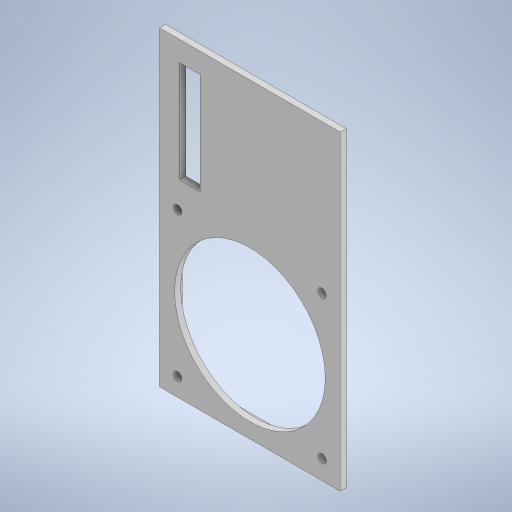
# Autodesk Inventor part: TapaControladora
Saved by Autodesk Inventor 2024 (Build 280153000, 153)
## iProperties
Created: 2023-11-28
Part Number: TapaControladora
Material: Genérico
Document SubType Name: Modeling
Designer: sergi
Density: 1 g/cm^3
Appearance: Valor por defecto
Author: sergi
Autodesk Inventor part; units mm, degrees
ref_plane "YZ Plane" through (0, 0, 0) normal (1, 0, 0) x (0, 1, 0)
ref_plane "XZ Plane" through (0, 0, 0) normal (0, 1, 0) x (-1, 0, 0)
ref_plane "XY Plane" through (0, 0, 0) normal (0, 0, 1) x (1, 0, 0)
sketch "Boceto1" plane through (0, 0, 0) normal (0, 0, 1) x (1, 0, 0)
  line L0 (-44.66, 76.85) -> (-44.66, -76.85) projected
  line L1 (-44.66, -76.85) -> (44.66, -76.85) projected
  line L2 (44.66, -76.85) -> (44.66, 76.85) projected
  line L3 (44.66, 76.85) -> (-44.66, 76.85) projected
  line L4 (41.66, -73.85) -> (-41.66, -73.85) projected
  line L5 (-41.66, -73.85) -> (-41.66, 73.85) projected
  line L6 (-41.66, 73.85) -> (41.66, 73.85) projected
  line L7 (41.66, 73.85) -> (41.66, -73.85) projected
  point P0 (0, 0)
extrude "Extrusión1" add sketch "Boceto1" along normal blind 3 contours L3 L2 L1 L0 | L4 L5 L6 L7
sketch "Boceto2" plane through (0, 0, 3) normal (0, 0, 1) x (1, 0, 0)
  line L0 (15.66, 13.175) -> (25.66, 13.175) projected
  line L1 (25.66, 13.175) -> (25.66, 9.175) projected
  line L2 (25.66, 9.175) -> (15.66, 9.175) projected
  line L3 (15.66, 9.175) -> (15.66, 13.175) projected
  line L4 (-21.66, 30.85) -> (-31.66, 30.85) projected
  line L5 (-31.66, 30.85) -> (-31.66, 34.85) projected
  line L6 (-31.66, 34.85) -> (-21.66, 34.85) projected
  line L7 (-21.66, 34.85) -> (-21.66, 30.85) projected
  line L8 (25.66, 30.85) -> (15.66, 30.85) projected
  line L9 (15.66, 30.85) -> (15.66, 34.85) projected
  line L10 (15.66, 34.85) -> (25.66, 34.85) projected
  line L11 (25.66, 34.85) -> (25.66, 30.85) projected
  line L12 (-31.66, 13.175) -> (-21.66, 13.175) projected
  line L13 (-21.66, 13.175) -> (-21.66, 9.175) projected
  line L14 (-21.66, 9.175) -> (-31.66, 9.175) projected
  line L15 (-31.66, 9.175) -> (-31.66, 13.175) projected
  circle A0 centre (32.34, 65.85) radius 4.5 projected
  circle A1 centre (-33.66, 39.85) radius 4.5 projected
  line L16 (38.16, -57.55) -> (38.16, -73.85) projected
  line L17 (38.16, -73.85) -> (41.66, -73.85) projected
  line L18 (41.66, -73.85) -> (41.66, 73.85) projected
  line L19 (41.66, 73.85) -> (-41.66, 73.85) projected
  line L20 (-41.66, 73.85) -> (-41.66, -73.85) projected
  line L21 (-41.66, -73.85) -> (23.76, -73.85) projected
  circle A2 centre (32.34, 39.85) radius 4.5 projected
  circle A3 centre (-33.66, 65.85) radius 4.5 projected
  line L22 (-44.66, 76.85) -> (-44.66, -76.85) projected
  line L23 (-44.66, 76.85) -> (-44.66, -76.85) projected
  line L24 (-44.66, -76.85) -> (44.66, -76.85) projected
  line L25 (44.66, -76.85) -> (44.66, 76.85) projected
  line L26 (44.66, 76.85) -> (-44.66, 76.85) projected
  line L27 (-44.66, 76.85) -> (-44.66, -76.85) projected
  line L28 (-41.66, -73.85) -> (41.66, -73.85)
  line L29 (41.66, -73.85) -> (41.66, 73.85)
  line L30 (41.66, 73.85) -> (-41.66, 73.85)
  line L31 (-41.66, 73.85) -> (-41.66, -73.85)
  line L32 (-41.66, -73.85) -> (41.66, -73.85)
  line L33 (41.66, -73.85) -> (41.66, 9.47)
  line L34 (41.66, 9.47) -> (-41.66, 9.47)
  line L35 (-41.66, 9.47) -> (-41.66, -73.85)
  line L36 (40, 7.81) -> (-40, 7.81)
  line L37 (-40, 7.81) -> (-40, -72.19)
  line L38 (-40, -72.19) -> (40, -72.19)
  line L39 (40, -72.19) -> (40, 7.81)
  line L40 (40, 7.81) -> (-40, -72.19) construction
  line L41 (-40, 7.81) -> (40, -72.19) construction
  line L42 (-37.8, -69.99) -> (-37.8, 5.61)
  line L43 (-37.8, 5.61) -> (37.8, 5.61)
  line L44 (37.8, 5.61) -> (37.8, -69.99)
  line L45 (37.8, -69.99) -> (-37.8, -69.99)
  circle A4 centre (-35.7, -67.89) radius 2.1
  circle A5 centre (0, -32.19) radius 37.25
  circle A6 centre (-35.7, 3.51) radius 2.1
  circle A7 centre (35.7, 3.51) radius 2.1
  circle A8 centre (35.7, -67.3145) radius 2.1
  point P0 (0, 0)
  dimension "d9" = 83.32
  dimension "d10" = 83.32
  dimension "d11" = 83.32
  dimension "d12" = 80
  dimension "d13" = 80
  dimension "d14" = 2.2
  dimension "d15" = 4.2
  dimension "d16" = 74.5
  dimension "d17" = 4.2
  dimension "d18" = 4.2
  dimension "d19" = 4.2
  constraints: 36 end point, 8 parallel, 7 tangent, 5 centre point, 4 perpendicular, 3 horizontal, 2 midpoint, 1 coincident, 3 other
  measures "d9" distance between parallel lines of L18 L31
  measures "d10" distance of L34.end L33.end
  measures "d11" distance of L33.end L32.end
  measures "d12" distance of L38.end L37.end
  measures "d13" distance of L37.end L36.end
  measures "d14" distance between parallel lines of L37 L42
  measures "d15" diameter of A4
  measures "d16" diameter of A5
  measures "d17" diameter of A6
  measures "d18" diameter of A7
  measures "d19" diameter of A8
sketch "Boceto3" plane through (0, 0, 0) normal (0, 0, -1) x (-1, 0, 0)
  line L0 (-44.66, -76.85) -> (-44.66, 76.85) projected
  line L1 (-44.66, -76.85) -> (-44.66, 76.85) projected
  line L2 (-41.66, 73.85) -> (-41.66, -73.85) projected
  line L3 (-41.66, -73.85) -> (41.66, -73.85) projected
  line L4 (41.66, -73.85) -> (41.66, 73.85) projected
  line L5 (41.66, 73.85) -> (-41.66, 73.85) projected
  line L6 (-41.66, -73.85) -> (41.66, -73.85)
  line L7 (41.66, -73.85) -> (41.66, 73.85)
  line L8 (41.66, 73.85) -> (-41.66, 73.85)
  line L9 (-41.66, 73.85) -> (-41.66, -73.85)
  line L10 (-41.41, 73.6) -> (-41.41, -73.6)
  line L11 (-41.41, -73.6) -> (41.41, -73.6)
  line L12 (41.41, -73.6) -> (41.41, 73.6)
  line L13 (41.41, 73.6) -> (-41.41, 73.6)
  line L14 (39.41, -71.6) -> (-39.41, -71.6)
  line L15 (-39.41, -71.6) -> (-39.41, 71.6)
  line L16 (-39.41, 71.6) -> (39.41, 71.6)
  line L17 (39.41, 71.6) -> (39.41, -71.6)
  point P0 (0, 0)
  dimension "d2" = 0.25
  dimension "d3" = 2
  constraints: 24 end point, 2 parallel, 1 horizontal, 1 perpendicular, 6 other
  measures "d2" distance between parallel lines of L5 L13
  measures "d3" distance between parallel lines of L11 L14
extrude "Extrusión2" add sketch "Boceto3" along normal blind 3 contours L13 L12 L11 L10
chamfer "Chaflán1" distance 1 angle 45 4 edges at (0, -73.6, -3) (41.41, 0, -3) (0, 73.6, -3) (-41.41, 0, -3) measured on face at (0, -73.1, -3) measured on face at (-40.91, 0, -3) measured on face at (40.91, 0, -3) measured on face at (0, 73.1, -3)
extrude "Extrusión3" cut sketch "Boceto2" against normal blind 3 contours A8 | A4 | A6 | A7 | A5
sketch "Boceto4" plane through (0, 0, 3) normal (0, 0, 1) x (1, 0, 0)
  circle A0 centre (35.7, 3.51) radius 2.1 projected
  circle A1 centre (35.7, -67.3145) radius 2.1 projected
  circle A2 centre (-35.7, 3.51) radius 2.1 projected
  circle A3 centre (-35.7, -67.89) radius 2.1 projected
  circle A4 centre (0, -32.19) radius 37.25 projected
  line L0 (-44.66, -76.85) -> (44.66, -76.85) projected
  line L1 (44.66, -76.85) -> (44.66, 76.85) projected
  line L2 (44.66, 76.85) -> (-44.66, 76.85) projected
  line L3 (-44.66, 76.85) -> (-44.66, -76.85) projected
  line L4 (-34.66, -66.85) -> (34.66, -66.85)
  line L5 (34.66, -66.85) -> (34.66, 66.85)
  line L6 (34.66, 66.85) -> (-34.66, 66.85)
  line L7 (-34.66, 66.85) -> (-34.66, -66.85)
  line L8 (-34.66, 66.85) -> (-24.66, 66.85)
  line L9 (-24.66, 66.85) -> (-24.66, 16.85)
  line L10 (-24.66, 16.85) -> (-34.66, 16.85)
  line L11 (-34.66, 16.85) -> (-34.66, 66.85)
  point P0 (0, 0)
  point P1 (-34.66, 16.85)
  dimension "d22" = 10
  dimension "d23" = 10
  dimension "d24" = 50
  constraints: 16 end point, 2 parallel, 1 horizontal, 1 perpendicular, 3 other
  measures "d22" distance between parallel lines of L3 L7
  measures "d23" distance of L9.end L10.end
  measures "d24" distance of L8.end L9.end
extrude "Extrusión4" cut sketch "Boceto4" against normal blind 10 contours L9 L10 L7 L6
